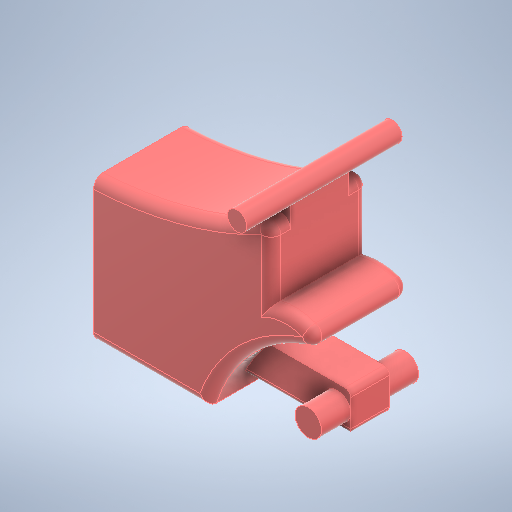
# Autodesk Inventor part: Moto
Saved by Autodesk Inventor 2025.2 (Build 292293000, 293)
## iProperties
Created: 2024-11-29
Part Number: Moto
Material: Plástico ABS
Document SubType Name: Modeling
Designer: usuario
Density: 1.06 g/cm^3
Appearance: Suave - Rojo
Author: usuario
Autodesk Inventor part; units mm, degrees
ref_plane "YZ Plane" through (0, 0, 0) normal (1, 0, 0) x (0, 1, 0)
ref_plane "XZ Plane" through (0, 0, 0) normal (0, 1, 0) x (-1, 0, 0)
ref_plane "XY Plane" through (0, 0, 0) normal (0, 0, 1) x (1, 0, 0)
sketch "Boceto1" plane through (0, 0, 0) normal (0, 0, 1) x (1, 0, 0)
  arc A0 (0, 10) -> (20, 10) centre (10, 27.5806) ccw
  arc A1 (22.8445, 5.4627) -> (16.6892, 0) centre (24.3208, -2.3999) ccw
  arc A2 (22.8445, 5.4627) -> (20, 6.2256) centre (20.7452, 3.3196) ccw
  arc A3 (3.5895, 0) -> (-1.3477, 5.3979) centre (-4.1292, -2.103) ccw
  arc A4 (0, 10) -> (-1.3477, 5.3979) centre (6.6508, 5.554) ccw
  line L0 (3.5895, 0) -> (16.6892, 0)
  line L1 (20, 6.2256) -> (20, 10)
  point P0 (0, 0)
  point P1 (10, 7.3549)
  point P2 (10, 10)
  dimension "d0" = 20
  dimension "d2" = 8
  dimension "d3" = 3
  dimension "d4" = 8
  dimension "d5" = 8
  constraints: 11 point on circle, 5 centre point, 4 end point, 1 horizontal, 1 perpendicular, 1 vertical alignment
  measures "d0" distance of A0.start L1.end
  measures "d2" radius of A1
  measures "d3" radius of A2
  measures "d4" radius of A3
  measures "d5" radius of A4
extrude "Extrusión1" add sketch "Boceto1" along normal blind 5
ref_plane "Plano de trabajo1" through (20, 10, 5) normal (-0.4944205, 0.8692228, 0) x (-0.8692228, -0.4944205, 0)
sketch "Boceto2" plane through (20, 10, 5) normal (-0.4944205, 0.8692228, 0) x (-0.8692228, -0.4944205, 0)
  circle A0 centre (1, -4) radius 0.5
  circle A1 centre (1, -1) radius 0.5
  line L0 (0, -5) -> (0, 0) projected
  line L1 (0, -5) -> (17.3845, -5) projected
  line L2 (0, 0) -> (17.3845, 0) projected
  point P0 (22.3287, -5)
  dimension "d8" = 1
  dimension "d9" = 1
  dimension "d10" = 1
  dimension "d11" = 1
  dimension "d12" = 1
  constraints: 2 centre point, 1 vertical alignment
  measures "d8" diameter of A0
  measures "d9" diameter of A1
  measures "d10" distance from line of L0 A0.centre
  measures "d11" distance from line of L1 A0.centre
  measures "d12" distance from line of L2 A1.centre
sketch3d "Boceto 3D1"
ref_plane "Plano de trabajo2" through (0, 0, 2.5) normal (0, 0, 1) x (1, 0, 0)
sketch "Boceto4" plane through (20, 6.2256, 0) normal (1, 0, 0) x (0, 0, -1)
  circle A0 centre (-2.5, -5.2256) radius 0.5
  line L0 (-5, -6.2256) -> (-5, -0.7628) projected
  line L1 (0, -6.2256) -> (-5, -6.2256) projected
  line L2 (0, -6.2256) -> (0, -0.7628) projected
  line L3 (-3.5, -3.2256) -> (-1.5, -3.2256)
  line L4 (-1.5, -3.2256) -> (-1.5, -5.2256)
  line L5 (-1.5, -5.2256) -> (-3.5, -5.2256)
  line L6 (-3.5, -5.2256) -> (-3.5, -3.2256)
  point P0 (-2.5, -6.2256)
  dimension "d20" = 1
  dimension "d21" = 1
  dimension "d22" = 2
  dimension "d23" = 2
  dimension "d24" = 1
  constraints: 8 end point, 2 midpoint, 2 parallel, 2 vertical alignment, 1 centre point, 1 horizontal, 1 perpendicular
  measures "d20" diameter of A0
  measures "d21" distance from line of A0.centre L1
  measures "d22" distance of L4.end L5.end
  measures "d23" distance of L3.end L4.end
  measures "d24" distance between parallel lines of L1 L5
extrude "Extrusión2" add sketch "Boceto4" along normal blind 2.6 and the other way blind 22.3 contours L5 A0 | A0 L5 L6 L3 L4 picked at (-2.3752, -5.1151)
fillet "Empalme1" radius 0.5 18 edges at (10, 7.3549, 5) (10, 7.3549, 0) (10.1393, 0, 5) (10.1393, 0, 0) (1.774, 3.2963, 0) (19.0105, 3.5836, 0) (19.0105, 3.5836, 5) (0, 10, 2.5) (-1.0268, 7.8023, 5) (1.774, 3.2963, 5) (20, 8.1128, 5) (20, 8.1128, 0) (20, 10, 2.5) (22.8445, 5.4627, 2.5) (21.5223, 6.2172, 0) (21.5223, 6.2172, 5) (-1.0268, 7.8023, 0) (-1.3477, 5.3979, 2.5)
fillet "Empalme2" radius 0.3 9 edges at (19.8396, 1, 3.5) (19.8396, 1, 1.5) (0.4723, 1, 1.5) (-2.3, 1, 2.5) (-0.134, 3, 1.5) (-0.134, 3, 3.5) (0.4723, 1, 3.5) (22.6, 3, 2.5) (22.6, 1, 2.5)
fillet "Empalme3" radius 0.3 1 edges at (-2.3, 3, 2.5)
sketch "Boceto7" plane through (17.2277, 1.3, 3.5) normal (0, 0, 1) x (1, 0, 0)
  circle A0 centre (4.6923, 0.7) radius 0.68
  line L0 (5.3723, 1.4) -> (5.3723, 0) projected
  line L1 (1.1904, 1.7) -> (5.0723, 1.7) projected
  point P0 (-17.2277, -1.3)
  point P1 (5.3723, 0.7)
  point P2 (5.3723, 0.7)
  dimension "d43" = 1.36
  constraints: 2 horizontal alignment, 2 midpoint, 2 other
extrude "Extrusión5" add sketch "Boceto7" along normal blind 1.5 and the other way blind 3.5
sketch "Boceto8" plane through (-2, 1.3, 3.5) normal (0, 0, 1) x (1, 0, 0)
  circle A0 centre (0.68, 0.7) radius 0.68
  line L0 (-0.3, 1.4) -> (-0.3, 0) projected
  line L1 (4.0319, 1.7) -> (0, 1.7) projected
  line L2 (0, 0) -> (0, 1.4) projected
  point P0 (2, -1.3)
  point P1 (0, 0.7)
  point P2 (0, 0.7)
  dimension "d48" = 1.36
  constraints: 2 horizontal alignment, 2 midpoint, 2 other
extrude "Extrusión6" add sketch "Boceto8" along normal blind 1.5 and the other way blind 3.5
ref_plane "Plano de trabajo3" through (8.85, 6.2256, 4.5) normal (1, 0, 0) x (0, 0, -1)
sketch "Boceto9" plane through (8.85, 6.2256, 4.5) normal (1, 0, 0) x (0, 0, -1)
  line L0 (7.2025, 6.1984) -> (-3.1783, 6.1984)
  line L1 (-3.1783, 6.1984) -> (-3.1783, -6.6541)
  line L2 (-3.1783, -6.6541) -> (7.2025, -6.6541)
  line L3 (7.2025, -6.6541) -> (7.2025, 6.1984)
  point P0 (4.5, -6.2256)
  constraints: 8 end point, 2 parallel, 1 horizontal, 1 perpendicular
extrude "Extrusión7" cut sketch "Boceto9" along normal blind 2 and the other way blind 20
ref_plane "Plano de trabajo4" through (0, 0, 2.5) normal (0, 0, -1) x (-1, 0, 0)
sketch "Boceto11" plane through (0, 0, 2.5) normal (0, 0, -1) x (-1, 0, 0)
  line L0 (-9.85, 21.5) -> (-32.35, 21.5)
  line L1 (-32.35, 21.5) -> (-32.35, -1)
  line L2 (-32.35, -1) -> (-9.85, -1)
  line L3 (-9.85, -1) -> (-9.85, 21.5)
  line L4 (-10.85, 6.8724) -> (-10.85, 0.5) projected
  line L5 (-10.85, 0) -> (-16.6892, 0) projected
  point P0 (0, 0)
  point P1 (-21.1, -1)
  dimension "d65" = 22.5
  dimension "d66" = 22.5
  dimension "d67" = 1
  dimension "d68" = 1
  constraints: 8 end point, 2 parallel, 1 horizontal, 1 midpoint, 1 perpendicular
  measures "d65" distance of L0.end L1.end
  measures "d66" distance of L0.start L0.end
  measures "d67" distance between parallel lines of L4 L3
  measures "d68" distance from line of point (-21.1, -1) L5
sketch "Boceto12" plane through (0, 0, 5) normal (0, 0, 1) x (1, 0, 0)
  arc A0 (20, 9.1604) -> (19.2708, 9.6048) centre (19.5, 9.1604) ccw projected
  circle A1 centre (19.75, 10.6604) radius 0.5
  line L0 (19.5, 9.1604) -> (20, 9.1604) projected
  point P0 (0, 0)
  dimension "d69" = 1
  dimension "d70" = 1.5
  dimension "d71" = 0.25
  constraints: 1 centre point
  measures "d69" diameter of A1
  measures "d70" distance from line of L0 A1.centre
  measures "d71" horizontal distance of A1.centre L0.start
extrude "Extrusión9" add sketch "Boceto12" along normal blind 1.5 and the other way blind 6.5
sketch "Boceto13" plane through (0, 0, 5) normal (0, 0, 1) x (1, 0, 0)
  point P0 (0, 0)
ref_plane "Plano de trabajo5" through (0, 0, 2.5) normal (0, 0, 1) x (1, 0, 0)
sketch "Boceto14" plane through (0, 0, 2.5) normal (0, 0, 1) x (1, 0, 0)
  arc A0 (20, 9.1604) -> (19.2708, 9.6048) centre (19.5, 9.1604) ccw projected
  line L0 (19.5, 9.1604) -> (20, 9.1604) projected
  line L1 (19.2708, 9.6048) -> (19.5, 9.1604) projected
  line L2 (19.5, 9.1604) -> (19.5, 10.2274)
  circle A1 centre (19.75, 10.6604) radius 0.5 projected
  line L3 (20, 9.1604) -> (20, 10.2274)
  point P0 (0, 0)
  point P1 (19.5, 9.6604)
  constraints: 4 end point, 2 point on circle, 1 vertical
extrude "Extrusión10" add sketch "Boceto14" along normal mid plane 3 contours A0 L2 A1 L3
scale "Escala1" factors (6, 6, 6) then translate (-67.9518, -2.5, 0) bodies 1
